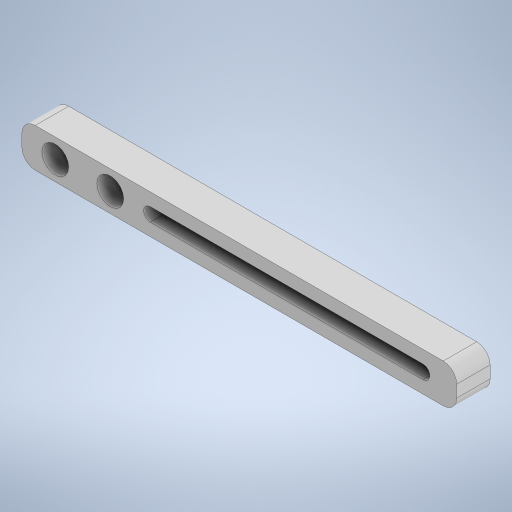
# Autodesk Inventor part: Locking Lever
Saved by Autodesk Inventor 2024 (Build 280153000, 153)
## iProperties
Created: 2024-09-25
Part Number: Locking Lever
Material: Generic
Document SubType Name: Modeling
Designer: Kemper Room 121
Density: 1 g/cm^3
Appearance: Default
Author: Kemper Room 121
Autodesk Inventor part; units mm, degrees
ref_plane "YZ Plane" through (0, 0, 0) normal (1, 0, 0) x (0, 1, 0)
ref_plane "XZ Plane" through (0, 0, 0) normal (0, 1, 0) x (-1, 0, 0)
ref_plane "XY Plane" through (0, 0, 0) normal (0, 0, 1) x (1, 0, 0)
sketch "Sketch1" plane through (0, 0, 0) normal (0, 0, 1) x (1, 0, 0)
  line L0 (0, 0) -> (65, 0)
  line L1 (65, 0) -> (65, 5.8)
  line L2 (65, 5.8) -> (0, 5.8)
  line L3 (0, 5.8) -> (0, 0)
  line L4 (0, 0) -> (0, 2.9)
  line L5 (0, 2.9) -> (5, 2.9)
  line L6 (5, 2.9) -> (13.2178, 2.9)
  circle A0 centre (5, 2.9) radius 1
  circle A1 centre (13.2178, 2.9) radius 1
  line L7 (13.2178, 2.9) -> (19.2178, 2.9)
  line L8 (19.2178, 2.9) -> (60, 2.9)
  circle A2 centre (19.2178, 2.9) radius 1
  circle A3 centre (60, 2.9) radius 1
  line L9 (19.2178, 3.9) -> (60, 3.9)
  line L10 (60, 1.9) -> (19.2178, 1.9)
  point P0 (65, 2.9)
  dimension "d0" = 65
  dimension "d1" = 5.8
  dimension "d2" = 2.9
  dimension "d3" = 5
  dimension "d4" = 8.2178
  dimension "d5" = 2
  dimension "d6" = 2
  dimension "d7" = 6
  dimension "d8" = 5
  dimension "d9" = 2
  dimension "d10" = 2
  constraints: 22 end point, 4 centre point, 4 coincident, 4 perpendicular, 4 point on circle, 3 horizontal, 2 midpoint, 2 tangent, 1 point on line
  measures "d0" distance of L0.start L0.end
  measures "d1" distance of L2.end L0.start
  measures "d2" distance of L0.start L4.end
  measures "d3" distance of L4.end L5.end
  measures "d4" distance of L5.end L6.end
  measures "d5" diameter of A0
  measures "d6" diameter of A1
  measures "d7" distance of L7.start L7.end
  measures "d8" distance of point (65, 2.9) L8.end
  measures "d9" diameter of A2
  measures "d10" diameter of A3
extrude "Extrusion1" add sketch "Sketch1" along normal blind 5
fillet "Fillet1" radius 2 4 edges at (0, 5.8, 2.5) (65, 5.8, 2.5) (65, 0, 2.5) (0, 0, 2.5)
sketch "Sketch2" plane through (0, 0, 5) normal (0, 0, 1) x (1, 0, 0)
  arc A0 (0, 2) -> (2, 0) centre (2, 2) ccw projected
  line L0 (2, 0) -> (63, 0) projected
  arc A1 (63, 0) -> (65, 2) centre (63, 2) ccw projected
  line L1 (65, 2) -> (65, 3.8) projected
  arc A2 (65, 3.8) -> (63, 5.8) centre (63, 3.8) ccw projected
  line L2 (63, 5.8) -> (2, 5.8) projected
  arc A3 (2, 5.8) -> (0, 3.8) centre (2, 3.8) ccw projected
  line L3 (0, 3.8) -> (0, 2) projected
  arc A4 (19.2178, 3.9) -> (19.2178, 1.9) centre (19.2178, 2.9) ccw projected
  line L4 (19.2178, 3.9) -> (60, 3.9) projected
  arc A5 (60, 1.9) -> (60, 3.9) centre (60, 2.9) ccw projected
  line L5 (60, 1.9) -> (19.2178, 1.9) projected
  circle A6 centre (13.2178, 2.9) radius 1 projected
  circle A7 centre (5, 2.9) radius 1 projected
  circle A8 centre (5, 2.9) radius 2
  circle A9 centre (13.2178, 2.9) radius 2
  point P0 (0, 0)
  dimension "d14" = 4
  dimension "d15" = 4
  constraints: 2 centre point, 2 coincident
  measures "d14" diameter of A8
  measures "d15" diameter of A9
extrude "Extrusion2" cut sketch "Sketch2" against normal blind 3 contours A7 | A8 | A9
equation "\"d2\" = 0.5 * d1"
equation "\"d6\" = d5"
equation "\"d7\" = d8 + 0.5 * d5"
equation "\"d9\" = d5"
equation "\"d10\" = d5"
equation "\"d15\" = d14"
body "Solid1"
